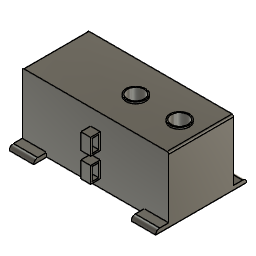
jpole uhf gövde (Autodesk Fusion 360 design; units mm, degrees)
Autodesk Fusion 360 part; units mm, degrees
sketch "Sketch3" plane through (0, 0, 0) normal (0, 0, 1) x (1, 0, 0)
  line L0 (-45, 20) -> (45, 20)
  line L1 (45, 20) -> (45, -20)
  line L2 (45, -20) -> (-45, -20)
  line L3 (-45, -20) -> (-45, 20)
  line L4 (-45, 20) -> (45, -20) construction
  line L5 (45, 20) -> (-45, -20) construction
  dimension "d7" = 90
  dimension "d8" = 40
  constraint horizontal L0
  constraint perpendicular L0 L1
  constraint parallel L0 L2
  constraint parallel L1 L3
  constraint coincident L4 origin
  constraint coincident L5 origin
  measures "d7" distance of L1.end L2.end
  measures "d8" distance of L0.end L1.end
extrude "Extrude2" add sketch "Sketch3" along normal blind 40
sketch "Sketch4" plane through (0, 0, 40) normal (0, 0, 1) x (-1, 0, 0)
  line L0 (45, 20) -> (-45, 20)
  line L1 (-45, 20) -> (-45, -20)
  line L2 (-45, -20) -> (45, -20)
  line L3 (45, -20) -> (45, 20)
  circle A0 centre (-4.8585, 0.0611) radius 5.95
  circle A1 centre (-31.8585, 0.0956) radius 5.95
  circle A2 centre (-4.8585, 0.0611) radius 5.2
  circle A3 centre (-31.8585, 0.0956) radius 5.2
  point P0 (-10.0585, 0.0565)
  point P1 (-26.6585, 0.0796)
  dimension "d11" = 11.9
  dimension "d12" = 11.9
  dimension "d24" = 10.4
  dimension "d25" = 10.4
  dimension "d142" = 16.6
  constraint concentric A0 A2
  constraint concentric A1 A3
  constraint coincident A2 P0
  constraint coincident A3 P1
  measures "d11" diameter of A0
  measures "d12" diameter of A1
  measures "d24" diameter of A2
  measures "d25" diameter of A3
  measures "d142" distance of P0 P1
extrude "Extrude36" add sketch "Sketch4" along normal blind 1 contours A0 | A1
shell "Shell3" thickness 2.5 removed faces 1 at (-15, 20, 13.3333)
extrude "Extrude5" add sketch "Sketch4" against normal blind 37.5 contours A0 | A1 | A2 | A3
extrude "Extrude6" cut sketch "Sketch4" against normal blind 37.5 contours A2 | A3
sketch "Sketch6" plane through (-45, 0, 0) normal (-1, 0, 0) x (0, -1, 0)
  line L0 (-20, 0) -> (20, 0)
  line L1 (20, 0) -> (20, 40)
  line L2 (20, 40) -> (-20, 40)
  line L3 (-20, 40) -> (-20, 0)
  circle A0 centre (0, 25) radius 8
  dimension "d33" = 16
  measures "d33" diameter of A0
extrude "Extrude8" cut sketch "Sketch6" against normal blind 5 contours A0
sketch "Sketch9" plane through (42.5, 0, 0) normal (-1, 0, 0) x (0, -1, 0)
  line L0 (-20, 2.5) -> (17.5, 2.5)
  line L1 (17.5, 2.5) -> (17.5, 37.5)
  line L2 (17.5, 37.5) -> (-20, 37.5)
  line L3 (-20, 37.5) -> (-20, 2.5)
  line L4 (-20, 37.5) -> (-14, 37.5)
  line L5 (-14, 37.5) -> (-14, 33.5)
  line L6 (-14, 33.5) -> (-20, 33.5)
  line L7 (-20, 33.5) -> (-20, 37.5)
  line L8 (-20, 2.5) -> (-14, 2.5)
  line L9 (-14, 2.5) -> (-14, 6.5)
  line L10 (-14, 6.5) -> (-20, 6.5)
  line L11 (-20, 6.5) -> (-20, 2.5)
  dimension "d64" = 6
  dimension "d65" = 4
  dimension "d66" = 4
  dimension "d67" = 6
  constraint horizontal L4
  constraint vertical L5
  constraint horizontal L6
  constraint vertical L7
  constraint coincident L2.end L3.start
  constraint horizontal L8
  constraint vertical L9
  constraint horizontal L10
  constraint vertical L11
  constraint coincident L0.start L3.end
  measures "d64" distance of L5.end L6.end
  measures "d65" distance of L4.end L5.end
  measures "d66" distance of L8.end L9.end
  measures "d67" distance of L9.end L10.end
extrude "Extrude12" add sketch "Sketch9" along normal blind 4 contours L0 L3 L8 L9 L10 L11 | L2 L3 L4 L5 L6 L7
sketch "Sketch10" plane through (-42.5, 0, 0) normal (1, 0, 0) x (0, 1, 0)
  circle A0 centre (0, 25) radius 8
  line L0 (-17.5, 2.5) -> (20, 2.5)
  line L1 (20, 2.5) -> (20, 37.5)
  line L2 (20, 37.5) -> (-17.5, 37.5)
  line L3 (-17.5, 37.5) -> (-17.5, 2.5)
  line L4 (20, 37.5) -> (14, 37.5)
  line L5 (14, 37.5) -> (14, 33.5)
  line L6 (14, 33.5) -> (20, 33.5)
  line L7 (20, 33.5) -> (20, 37.5)
  line L8 (20, 2.5) -> (14, 2.5)
  line L9 (14, 2.5) -> (14, 6.5)
  line L10 (14, 6.5) -> (20, 6.5)
  line L11 (20, 6.5) -> (20, 2.5)
  dimension "d47" = 6
  dimension "d48" = 4
  dimension "d49" = 6
  dimension "d50" = 4
  constraint horizontal L4
  constraint vertical L5
  constraint horizontal L6
  constraint vertical L7
  constraint coincident L1.end L2.start
  constraint horizontal L8
  constraint vertical L9
  constraint horizontal L10
  constraint vertical L11
  constraint coincident L0.end L1.start
  measures "d47" distance of L1.end L4.end
  measures "d48" distance of L1.end L6.end
  measures "d49" distance of L0.end L8.end
  measures "d50" distance of L0.end L10.end
extrude "Extrude13" add sketch "Sketch10" along normal blind 4 contours L0 L1 L8 L9 L10 L11 | L1 L2 L4 L5 L6 L7
sketch "Sketch11" plane through (0, 20, 0) normal (0, 1, 0) x (-1, 0, 0)
  line L0 (-42.5, 6.5) -> (-42.5, 33.5)
  line L1 (-42.5, 33.5) -> (-38.5, 33.5)
  line L2 (-38.5, 33.5) -> (-38.5, 37.5)
  line L3 (-38.5, 37.5) -> (38.5, 37.5)
  line L4 (38.5, 37.5) -> (38.5, 33.5)
  line L5 (38.5, 33.5) -> (42.5, 33.5)
  line L6 (42.5, 33.5) -> (42.5, 6.5)
  line L7 (42.5, 6.5) -> (38.5, 6.5)
  line L8 (38.5, 6.5) -> (38.5, 2.5)
  line L9 (38.5, 2.5) -> (-38.5, 2.5)
  line L10 (-38.5, 2.5) -> (-38.5, 6.5)
  line L11 (-38.5, 6.5) -> (-42.5, 6.5)
  line L12 (-45, 0) -> (45, 0)
  line L13 (45, 0) -> (45, 40)
  line L14 (45, 40) -> (-45, 40)
  line L15 (-45, 40) -> (-45, 0)
  line L16 (-45, 2.5) -> (-30, 2.5)
  line L17 (-30, 2.5) -> (-30, 0)
  line L18 (-30, 0) -> (-45, 0)
  line L19 (-45, 0) -> (-45, 2.5)
  line L20 (45, 0) -> (30, 0)
  line L21 (30, 0) -> (30, 2.5)
  line L22 (30, 2.5) -> (45, 2.5)
  line L23 (45, 2.5) -> (45, 0)
  dimension "d55" = 15
  dimension "d56" = 2.5
  dimension "d57" = 15
  dimension "d95" = 2.5
  constraint horizontal L16
  constraint vertical L17
  constraint horizontal L18
  constraint vertical L19
  constraint coincident L12 L17.end
  constraint coincident L15 L16.start
  constraint horizontal L20
  constraint vertical L21
  constraint horizontal L22
  constraint vertical L23
  constraint coincident L12.end L13.start
  measures "d55" distance of L12.end L20.end
  measures "d56" distance of L12.end L22.end
  measures "d57" distance of L16.start L16.end
  measures "d95" distance of L16.start L12.start
extrude "Extrude14" add sketch "Sketch11" along normal blind 8 contours L9 L12 L15 L16 L17 L18 L19
extrude "Extrude15" add sketch "Sketch11" along normal blind 8 contours L9 L12 L13 L20 L21 L22 L23
sketch "Sketch12" plane through (0, -20, 0) normal (0, -1, 0) x (1, 0, 0)
  line L0 (-45, 0) -> (45, 0)
  line L1 (45, 0) -> (45, 40)
  line L2 (45, 40) -> (-45, 40)
  line L3 (-45, 40) -> (-45, 0)
  line L4 (-45, 0) -> (-30, 0)
  line L5 (-30, 0) -> (-30, 2.5)
  line L6 (-30, 2.5) -> (-45, 2.5)
  line L7 (-45, 2.5) -> (-45, 0)
  line L8 (45, 0) -> (30, 0)
  line L9 (30, 0) -> (30, 2.5)
  line L10 (30, 2.5) -> (45, 2.5)
  line L11 (45, 2.5) -> (45, 0)
  dimension "d96" = 2.5
  dimension "d97" = 2.5
  constraint horizontal L4
  constraint vertical L5
  constraint horizontal L6
  constraint vertical L7
  constraint coincident L0.start L3.end
  constraint horizontal L8
  constraint vertical L9
  constraint horizontal L10
  constraint vertical L11
  constraint coincident L0.end L1.start
  measures "d96" distance of L4.end L5.end
  measures "d97" distance of L8.end L9.end
extrude "Extrude16" add sketch "Sketch12" along normal blind 8 contours L0 L3 L4 L5 L6 L7 | L0 L1 L8 L9 L10 L11
hole "Hole1" at (40.5479, 20, 35.8551) direction (0, -1, 0) diameter 3.2 depth 6 tip angle 180
hole "Hole2" at (40.662, 20, 4.4495) direction (0, -1, 0) diameter 3.2 depth 6 tip angle 118
hole "Hole4" at (-40.567, 20, 35.788) direction (0, -1, 0) diameter 3.2 depth 6 tip angle 180
hole "Hole5" at (-40.5957, 20, 4.4643) direction (0, -1, 0) diameter 3.2 depth 6 tip angle 180
ref_plane "WorkPlane1" through (0, 85, 0) normal (0, 1, 0) x (0, 0, 1)
sketch "Sketch21" plane through (0, 85, 0) normal (0, 1, 0) x (1, 0, 0)
  line L0 (45, -40) -> (-45, -40)
  line L1 (-45, -40) -> (-45, -3)
  line L2 (-45, -3) -> (45, -3)
  line L3 (45, -3) -> (45, -40)
  constraint horizontal L0
  constraint vertical L1
  constraint horizontal L2
  constraint vertical L3
fillet "Fillet1" radius 2.5 1 edges at (37.5, -28, 2.5)
fillet "Fillet2" radius 2.5 1 edges at (-37.5, -28, 2.5)
fillet "Fillet3" radius 2.5 1 edges at (37.5, 28, 2.5)
fillet "Fillet4" radius 2.5 1 edges at (-37.5, 28, 2.5)
extrude "Extrude19" add 1 faces at (-10, 20, 0.8333) along direction (0, 1, 0) blind 2
sketch "Sketch17" plane through (0, 0, 0) normal (0, 1, 0) x (1, 0, 0)
  line L0 (32, -3) -> (32, -20.3)
  circle A0 centre (32, -20.3) radius 1.75
  line L1 (4.8797, -3) -> (4.8797, -20.3)
  circle A1 centre (4.8797, -20.3) radius 1.75
  dimension "d107" = 17.3
  dimension "d108" = 3.5
  dimension "d109" = 17.3
  dimension "d110" = 3.5
  constraint vertical L0
  constraint coincident L0.end A0.centre
  constraint vertical L1
  constraint coincident L1.end A1.centre
  measures "d107" distance of L0.start L0.end
  measures "d108" diameter of A0
  measures "d109" distance of L1.start L1.end
  measures "d110" diameter of A1
extrude "Extrude21" cut sketch "Sketch17" along normal blind 17 contours A1
extrude "Extrude20" cut sketch "Sketch17" along normal blind 14 contours A0
fillet "Fillet5" radius 1 1 edges at (45, 0, 40)
fillet "Fillet6" radius 1 1 edges at (-45, 0, 40)
extrude "Extrude22" add 1 faces at (-38.5, 16, 36.1667) along direction (1, 0, 0) blind 1
extrude "Extrude23" add 1 faces at (-38.5, 16, 3.8333) along direction (1, 0, 0) blind 1
extrude "Extrude24" add 1 faces at (38.5, 18, 36.1667) along direction (-1, 0, 0) blind 1
extrude "Extrude25" add 1 faces at (38.5, 16, 3.8333) along direction (-1, 0, 0) blind 1
sketch "Sketch18" plane through (0, -17.5, 0) normal (0, 1, 0) x (-1, 0, 0)
  line L0 (-42.5, 2.5) -> (42.5, 2.5)
  line L1 (42.5, 2.5) -> (42.5, 37.5)
  line L2 (42.5, 37.5) -> (-42.5, 37.5)
  line L3 (-42.5, 37.5) -> (-42.5, 2.5)
sketch "Sketch19" plane through (0, 0, 2.5) normal (0, 0, 1) x (-1, 0, 0)
  line L0 (-37.5, -20) -> (-45, -20)
  line L1 (-45, -20) -> (-45, -25.5)
  line L2 (-45, -25.5) -> (-30, -25.5)
  line L3 (-30, -25.5) -> (-30, -22)
  line L4 (-30, -22) -> (30, -22)
  line L5 (30, -22) -> (30, -25.5)
  line L6 (30, -25.5) -> (45, -25.5)
  line L7 (45, -25.5) -> (45, -20)
  line L8 (45, -20) -> (37.5, -20)
  line L9 (37.5, -20) -> (37.5, -14)
  line L10 (37.5, -14) -> (42.5, -14)
  line L11 (42.5, -14) -> (42.5, 17.5)
  line L12 (42.5, 17.5) -> (-42.5, 17.5)
  line L13 (-42.5, 17.5) -> (-42.5, -14)
  line L14 (-42.5, -14) -> (-37.5, -14)
  line L15 (-37.5, -14) -> (-37.5, -20)
  circle A0 centre (-31.8585, 0.0956) radius 5.95
  circle A1 centre (-4.8585, 0.0611) radius 5.95
sketch "Sketch22" plane through (0, 20, 0) normal (0, 1, 0) x (-1, 0, 0)
  circle A0 centre (40.5957, 4.4643) radius 1.6
  circle A1 centre (40.567, 35.788) radius 1.6
  circle A2 centre (-40.662, 4.4495) radius 1.6
  circle A3 centre (-40.5479, 35.8551) radius 1.6
  arc A4 (45, 39) -> (44, 40) centre (44, 39) ccw
  line L0 (44, 40) -> (-44, 40)
  arc A5 (-44, 40) -> (-45, 39) centre (-44, 39) ccw
  line L1 (-45, 39) -> (-45, 2.5)
  line L2 (-45, 2.5) -> (-37.5, 2.5)
  line L3 (-37.5, 2.5) -> (-37.5, 6.5)
  line L4 (-37.5, 6.5) -> (-42.5, 6.5)
  line L5 (-42.5, 6.5) -> (-42.5, 33.5)
  line L6 (-42.5, 33.5) -> (-37.5, 33.5)
  line L7 (-37.5, 33.5) -> (-37.5, 37.5)
  line L8 (-37.5, 37.5) -> (37.5, 37.5)
  line L9 (37.5, 37.5) -> (37.5, 33.5)
  line L10 (37.5, 33.5) -> (42.5, 33.5)
  line L11 (42.5, 33.5) -> (42.5, 6.5)
  line L12 (42.5, 6.5) -> (37.5, 6.5)
  line L13 (37.5, 6.5) -> (37.5, 2.5)
  line L14 (37.5, 2.5) -> (45, 2.5)
  line L15 (45, 2.5) -> (45, 39)
  circle A6 centre (-40.5479, 35.8551) radius 1.6
  circle A7 centre (40.567, 35.788) radius 1.6
  circle A8 centre (40.5957, 4.4643) radius 1.6
  circle A9 centre (-40.662, 4.4495) radius 1.6
  constraint concentric A3 A6
  constraint concentric A1 A7
  constraint concentric A0 A8
  constraint concentric A2 A9
sketch "Sketch23" plane through (0, -20, 0) normal (0, -1, 0) x (1, 0, 0)
  arc A0 (-44, 40) -> (-45, 39) centre (-44, 39) ccw
  line L0 (-45, 39) -> (-45, 2.5)
  line L1 (-45, 2.5) -> (-30, 2.5)
  line L2 (-30, 2.5) -> (-30, 0)
  line L3 (-30, 0) -> (30, 0)
  line L4 (30, 0) -> (30, 2.5)
  line L5 (30, 2.5) -> (45, 2.5)
  line L6 (45, 2.5) -> (45, 39)
  arc A1 (45, 39) -> (44, 40) centre (44, 39) ccw
  line L7 (44, 40) -> (-44, 40)
  line L8 (-3, 30) -> (3, 30)
  line L9 (3, 30) -> (3, 20)
  line L10 (3, 20) -> (-3, 20)
  line L11 (-3, 20) -> (-3, 30)
  line L12 (-3, 30) -> (3, 20) construction
  line L13 (3, 30) -> (-3, 20) construction
  line L14 (-3, 15) -> (3, 15)
  line L15 (3, 15) -> (3, 5)
  line L16 (3, 5) -> (-3, 5)
  line L17 (-3, 5) -> (-3, 15)
  line L18 (-3, 15) -> (3, 5) construction
  line L19 (3, 15) -> (-3, 5) construction
  point P0 (0, 25)
  point P1 (0, 10)
  constraint horizontal L8
  constraint perpendicular L8 L9
  constraint parallel L8 L10
  constraint parallel L9 L11
  constraint coincident L12 P0
  constraint coincident L13 P0
  constraint horizontal L14
  constraint perpendicular L14 L15
  constraint parallel L14 L16
  constraint parallel L15 L17
  constraint coincident L18 P1
  constraint coincident L19 P1
extrude "Extrude33" add sketch "Sketch23" along normal blind 6 contours L14 L15 L16 L17
extrude "Extrude32" add sketch "Sketch23" along normal blind 6 contours L8 L9 L10 L11
sketch "Sketch24" plane through (-3, 0, 0) normal (-1, 0, 0) x (0, -1, 0)
  line L0 (20, 30) -> (20, 20)
  line L1 (20, 20) -> (26, 20)
  line L2 (26, 20) -> (26, 30)
  line L3 (26, 30) -> (20, 30)
  line L4 (25, 29) -> (21, 29)
  line L5 (21, 29) -> (21, 21)
  line L6 (21, 21) -> (25, 21)
  line L7 (25, 21) -> (25, 29)
  line L8 (25, 14) -> (21, 14)
  line L9 (21, 14) -> (21, 6)
  line L10 (21, 6) -> (25, 6)
  line L11 (25, 6) -> (25, 14)
  constraint horizontal L4
  constraint vertical L5
  constraint horizontal L6
  constraint vertical L7
  constraint horizontal L8
  constraint vertical L9
  constraint horizontal L10
  constraint vertical L11
extrude "Extrude34" cut sketch "Sketch24" against normal blind 24 contours L4 L5 L6 L7 | L8 L9 L10 L11
